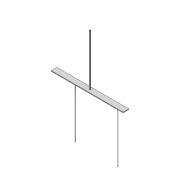
# Autodesk Inventor part: Part7
Saved by Autodesk Inventor 2017 (Build 210142000, 142)
## iProperties
Created: 2019-07-20
Part Number: Part7
Material: Generic
Document SubType Name: Modeling
Designer: Admin
Density: 1 g/cm^3
Appearance: Default
Author: Admin
Autodesk Inventor part; units mm, degrees
ref_plane "YZ Plane" through (0, 0, 0) normal (1, 0, 0) x (0, 1, 0)
ref_plane "XZ Plane" through (0, 0, 0) normal (0, 1, 0) x (-1, 0, 0)
ref_plane "XY Plane" through (0, 0, 0) normal (0, 0, 1) x (1, 0, 0)
sketch "Sketch1" plane through (0, 0, 0) normal (0, 0, 1) x (1, 0, 0)
  line L0 (4.4177, -4.0601) -> (-4.4177, -4.0601)
  line L1 (-4.4177, -4.0601) -> (-4.4177, 4.0601)
  line L2 (-4.4177, 4.0601) -> (4.4177, 4.0601)
  line L3 (4.4177, 4.0601) -> (4.4177, -4.0601)
  line L4 (4.4177, -4.0601) -> (-4.4177, 4.0601) construction
  line L5 (-4.4177, -4.0601) -> (4.4177, 4.0601) construction
  point P0 (0, 0)
  constraints: 12 end point, 2 parallel, 1 horizontal, 1 perpendicular
extrude "Extrusion1" add sketch "Sketch1" along normal blind 650
fillet "Fillet2" radius 3.25 4 edges at (0, 4.0601, 650) (-4.4177, 0, 650) (0, -4.0601, 650) (4.4177, 0, 650)
ref_plane "Work Plane1" through (4.4177, 0, 646.75) normal (0, 1, 0) x (1, 0, 0)
sketch "Sketch2" plane through (4.4177, 0, 646.75) normal (0, 1, 0) x (1, 0, 0)
  line L0 (-8.8354, 0) -> (0, 0) projected
  arc A0 (-8.8354, 0) -> (0, 0) centre (-4.4177, 1.3775) ccw
  line L1 (-8.8354, 0) -> (-8.8354, -4.2008)
  line L2 (-8.8354, -4.2008) -> (-4.4177, -4.2008)
  line L3 (-4.4177, -4.2008) -> (-4.4177, -3.25)
  point P0 (-4.4177, 646.75)
  constraints: 6 end point, 3 point on circle, 1 centre point, 1 perpendicular, 1 vertical
extrude "Extrusion2" cut sketch "Sketch2" along normal mid plane 20 contours L0 A0
sketch "Sketch3" plane through (4.4177, 4.0601, 646.75) normal (0, 1, 0) x (1, 0, 0)
  line L0 (-9.2871, 0) -> (1.4537, 0)
  line L1 (1.4537, 0) -> (1.4537, -3.6122)
  line L2 (1.4537, -3.6122) -> (-9.2871, -3.6122)
  line L3 (-9.2871, -3.6122) -> (-9.2871, 0)
  point P0 (-4.4177, 646.75)
  constraints: 8 end point, 2 parallel, 1 horizontal, 1 perpendicular
extrude "Extrusion3" cut sketch "Sketch3" against normal blind 25.5
sketch "Sketch4" plane through (4.4177, 4.0601, 646.75) normal (0, 1, 0) x (1, 0, 0)
  line L0 (-8.8354, 0) -> (0, 0) projected
  arc A0 (-8.8354, 0) -> (0, 0) centre (-4.4177, 0.2318) ccw
  point P0 (-4.4177, 646.75)
  constraints: 2 point on circle, 1 centre point
extrude "Extrusion4" add sketch "Sketch4" against normal blind 8.25
sketch "Sketch5" plane through (0, 0, 0) normal (0, 0, -1) x (-1, 0, 0)
  line L0 (-450, 35) -> (450, 35)
  line L1 (450, 35) -> (450, -35)
  line L2 (450, -35) -> (-450, -35)
  line L3 (-450, -35) -> (-450, 35)
  line L4 (-450, 35) -> (450, -35) construction
  line L5 (450, 35) -> (-450, -35) construction
  circle A0 centre (184.0275, 0) radius 5
  circle A1 centre (-350, 0) radius 5
  point P0 (0, 0)
  dimension "d11" = 900
  dimension "d12" = 70
  dimension "d14" = 10
  constraints: 12 end point, 2 centre point, 2 midpoint, 2 parallel, 1 horizontal, 1 perpendicular
  measures "d11" distance of L1.end L2.end
  measures "d12" distance of L0.end L1.end
  measures "d14" diameter of A0
extrude "Extrusion5" add sketch "Sketch5" along normal blind 10
extrude "Extrusion6" add sketch "Sketch5" along normal blind 658.25 contours A0 | A1
body "Solid1"
